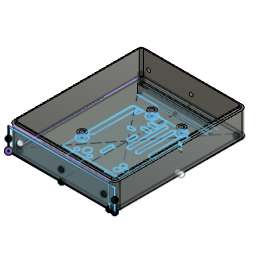
Toolbox-bottom (Autodesk Fusion 360 design; units mm, degrees)
Autodesk Fusion 360 part; units mm, degrees
sketch "Sketch1" plane through (0, 0, 0) normal (0, 1, 0) x (1, 0, 0)
  line L0 (5, 0) -> (95, 0)
  line L1 (100, 5) -> (100, 120)
  line L2 (95, 125) -> (5, 125)
  line L3 (0, 120) -> (0, 5)
  arc A0 (5, 125) -> (0, 120) centre (5, 120) ccw
  arc A1 (100, 120) -> (95, 125) centre (95, 120) ccw
  arc A2 (95, 0) -> (100, 5) centre (95, 5) ccw
  arc A3 (0, 5) -> (5, 0) centre (5, 5) ccw
  line L4 (5, 3) -> (95, 3)
  arc A4 (95, 3) -> (97, 5) centre (95, 5) ccw
  line L5 (97, 5) -> (97, 120)
  arc A5 (97, 120) -> (95, 122) centre (95, 120) ccw
  line L6 (95, 122) -> (5, 122)
  arc A6 (5, 122) -> (3, 120) centre (5, 120) ccw
  line L7 (3, 120) -> (3, 5)
  arc A7 (3, 5) -> (5, 3) centre (5, 5) ccw
  point P0 (100, 0)
  point P1 (0, 125)
  dimension "d1" = 100
  dimension "d2" = 125
  dimension "d5" = -3
  dimension "d9" = 5
  dimension "d10" = 5
  dimension "d11" = 5
  dimension "d12" = 5
  constraint horizontal L0
  constraint vertical L1
  constraint horizontal L2
  constraint vertical L3
  constraint coincident P1 L3
  constraint coincident P1 L2
  constraint tangent L3 A0
  constraint tangent L2 A0
  constraint tangent L2 A1
  constraint tangent L1 A1
  constraint coincident P0 L0
  constraint coincident P0 L1
  constraint tangent L0 A2
  constraint tangent L1 A2
  constraint coincident origin L3
  constraint coincident origin L0
  constraint tangent L3 A3
  constraint tangent L0 A3
  measures "d1" distance of origin P0
  measures "d2" distance of origin P1
  measures "d9" radius of A0
  measures "d10" radius of A1
  measures "d11" radius of A2
  measures "d12" radius of A3
extrude "Extrude1" add sketch "Sketch1" along normal blind 25 contours L0 L1 L2 L3 A0 A1 A2 A3 | L4 A4 L5 A5 L6 A6 L7 A7
extrude "Extrude2" cut sketch "Sketch1" along normal up to surface (23 mm away) from surface at 2 contours L4 A4 L5 A5 L6 A6 L7 A7
ref_plane "WorkPlane1" through (50, 12.5, -62.5) normal (0, 0, 1) x (1, 0, 0)
sketch "Sketch2" plane through (50, 10, -62.5) normal (0, 0, 1) x (1, 0, 0)
ref_plane "WorkPlane2" through (50, 13.5, -64) normal (0, 0, -1) x (-1, 0, 0)
ref_plane "WorkPlane3" through (50, 12.5, -62.5) normal (0, 0, 1) x (1, 0, 0)
sketch "Sketch4" plane through (50, 10, -62.5) normal (0, 0, 1) x (1, 0, 0)
  line L0 (50, 10) -> (50, 8)
  line L1 (50, 8) -> (48, 8)
  line L2 (48, 8) -> (48, 10)
  line L3 (48, 10) -> (50, 10)
  line L4 (50, -10) -> (47, -10)
  line L5 (50, 15) -> (48, 15)
  line L6 (48, 15) -> (48, 13)
  line L7 (48, 13) -> (50, 13)
  line L8 (50, 13) -> (50, 15)
  dimension "d29" = 2
  dimension "d53" = 2
  dimension "d54" = 2
  dimension "d55" = 2
  constraint perpendicular L0 L1
  constraint perpendicular L1 L2
  constraint perpendicular L0 L3
  constraint horizontal L4
  constraint horizontal L5
  constraint vertical L6
  constraint horizontal L7
  constraint vertical L8
  measures "d29" distance of L0 L2
  measures "d53" distance of L1 L3
  measures "d54" distance of L5.start L5.end
  measures "d55" distance of L5.start L7.end
sweep "Sweep1" cut profiles "Sketch4" along 8 edges at (1.4645, 25, -123.5355) (0, 25, -62.5) (1.4645, 25, -1.4645) (50, 25, 0) (98.5355, 25, -1.4645) (100, 25, -62.5) (98.5355, 25, -123.5355) (50, 25, -125) section 1 contours L5 L6 L7 L8
sketch "Sketch5" plane through (0, 0, 0) normal (0, 0, 1) x (1, 0, 0)
  line L0 (5, 23) -> (5, 0)
  line L1 (5, 0) -> (95, 0)
  line L2 (95, 0) -> (95, 23)
  line L3 (0, 0) -> (100, 0)
  line L4 (100, 0) -> (100, 20)
  line L5 (100, 20) -> (0, 20)
  line L6 (0, 20) -> (0, 0)
  circle A0 centre (11, 12) radius 1.75
  line L7 (95, 20) -> (95, 0)
  line L8 (95, 23) -> (5, 23)
  dimension "d19" = 3.5
  constraint horizontal L3
  constraint vertical L4
  constraint horizontal L5
  constraint vertical L6
  constraint coincident L3.start L6.end
  constraint coincident L5 L7.start
  constraint coincident L1.end L2.start
  measures "d19" diameter of A0
sketch "Sketch6" plane through (0, 0, 0) normal (0, 0, 1) x (1, 0, 0)
  line L0 (0, 0) -> (100, 0)
  line L1 (100, 0) -> (100, 20)
  line L2 (100, 20) -> (0, 20)
  line L3 (0, 20) -> (0, 0)
  line L4 (0, 0) -> (100, 0)
  line L5 (0, 0) -> (100, 0)
  line L6 (100, 0) -> (100, 20)
  line L7 (100, 20) -> (0, 20)
  line L8 (0, 20) -> (0, 0)
  circle A0 centre (50, 10) radius 1.75
  circle A1 centre (10, 10) radius 1.75
  circle A2 centre (90, 10) radius 1.75
  point P0 (0, 10)
  point P1 (100, 10)
  point P2 (50, 0)
  dimension "d20" = 20
  dimension "d21" = 100
  dimension "d22" = 3.5
  dimension "d23" = 3.5
  dimension "d24" = 3.5
  dimension "d25" = 10
  dimension "d26" = 10
  constraint horizontal L0
  constraint vertical L1
  constraint horizontal L2
  constraint vertical L3
  constraint coincident L0.start L3.end
  constraint horizontal L5
  constraint vertical L6
  constraint horizontal L7
  constraint vertical L8
  constraint midpoint L3 P0
  constraint midpoint L1 P1
  constraint midpoint L4 P2
  constraint vertical P2 A0.centre
  constraint horizontal P0 A0.centre
  constraint horizontal P0 A1.centre
  constraint horizontal P1 A2.centre
  measures "d20" distance of L1.end L0.end
  measures "d21" distance of L1.end L2.end
  measures "d22" diameter of A0
  measures "d23" diameter of A1
  measures "d24" diameter of A2
  measures "d25" distance of L3 A1.centre
  measures "d26" distance of L1 A2.centre
extrude "Extrude3" cut sketch "Sketch6" against normal up to surface (125 mm away) contours A0 | A1 | A2
sketch "nookduino_holes_thmt_fmsu" plane through (0, 2, 0) normal (0, 1, 0) x (1, 0, 0)
  spline S0 degree 3 poles (36.3365, 93.969) (36.3715, 93.969) (36.3998, 93.9972) (36.3998, 94.0324) (36.3998, 94.0672) (36.3715, 94.0958) (36.3365, 94.0958) knots 0 0 0 0 1 1 1 2 2 2 2
  spline S1 degree 3 poles (23.3685, 92.5565) (23.3437, 92.532) (23.3437, 92.4917) (23.3685, 92.4669) knots 0 0 0 0 1 1 1 1
  spline S2 degree 3 poles (23.3685, 92.4669) (23.3931, 92.4425) (23.4333, 92.4425) (23.4579, 92.4669) knots 1 1 1 1 2 2 2 2
  line L0 (73.3326, 26.3498) -> (73.3326, 28.0274)
  spline S3 degree 3 poles (44.503, 21.7606) (44.5381, 21.7606) (44.5664, 21.789) (44.5664, 21.824) (44.5664, 21.8591) (44.5381, 21.8874) (44.503, 21.8874) knots 0 0 0 0 1 1 1 2 2 2 2
  line L1 (23.4131, 92.5121) -> (24.9336, 94.0324)
  line L2 (38.8704, 96.5663) -> (71.5587, 96.5663)
  spline S4 degree 3 poles (38.617, 39.0459) (40.2416, 39.0459) (41.5581, 37.7292) (41.5581, 36.105) knots 0 0 0 0 1 1 1 1
  line L3 (41.5581, 36.105) -> (41.5581, 35.1974)
  spline S5 degree 3 poles (41.5581, 35.1974) (41.5581, 33.573) (40.2416, 32.2563) (38.617, 32.2563) knots 2 2 2 2 3 3 3 3
  spline S6 degree 3 poles (38.617, 32.2563) (36.9928, 32.2563) (35.6759, 33.573) (35.6759, 35.1974) knots 4 4 4 4 5 5 5 5
  line L4 (35.6759, 35.1974) -> (35.6759, 36.105)
  spline S7 degree 3 poles (35.6759, 36.105) (35.6759, 37.7292) (36.9928, 39.0459) (38.617, 39.0459) knots 6 6 6 6 7 7 7 7
  arc A0 (36.2917, 94.0772) -> (36.2917, 93.9876) centre (36.3364, 94.0324) ccw
  spline S8 degree 3 poles (36.2917, 93.9876) (36.3164, 93.9625) (36.3565, 93.9625) (36.3813, 93.9876) knots 1 1 1 1 2 2 2 2
  spline S9 degree 3 poles (76.5634, 28.149) (76.5634, 28.1141) (76.5916, 28.0856) (76.6264, 28.0856) (76.6616, 28.0856) (76.6898, 28.1141) (76.6898, 28.149) knots 0 0 0 0 1 1 1 2 2 2 2
  spline S10 degree 3 poles (24.9336, 94.0958) (24.8986, 94.0958) (24.8704, 94.0672) (24.8704, 94.0324) (24.8704, 93.9972) (24.8986, 93.969) (24.9336, 93.969) knots 0 0 0 0 1 1 1 2 2 2 2
  line L5 (44.503, 21.824) -> (44.503, 28.0856)
  arc A1 (38.9152, 96.5215) -> (38.9152, 96.611) centre (38.8706, 96.5663) ccw
  spline S11 degree 3 poles (38.9152, 96.611) (38.8906, 96.6358) (38.8504, 96.6358) (38.8258, 96.611) knots 1 1 1 1 2 2 2 2
  spline S12 degree 3 poles (43.0869, 75.547) (43.8496, 75.547) (44.4678, 74.9286) (44.4678, 74.1659) knots 0 0 0 0 1 1 1 1
  spline S13 degree 3 poles (44.4678, 74.1659) (44.4678, 73.4035) (43.8496, 72.7851) (43.0869, 72.7851) knots 2 2 2 2 3 3 3 3
  line L6 (43.0869, 72.7851) -> (40.0261, 72.7851)
  spline S14 degree 3 poles (40.0261, 72.7851) (39.2635, 72.7851) (38.6451, 73.4035) (38.6451, 74.1659) knots 4 4 4 4 5 5 5 5
  spline S15 degree 3 poles (38.6451, 74.1659) (38.6451, 74.9286) (39.2635, 75.547) (40.0261, 75.547) knots 6 6 6 6 7 7 7 7
  line L7 (40.0261, 75.547) -> (43.0869, 75.547)
  line L8 (36.3365, 94.0324) -> (38.8704, 96.5663)
  spline S16 degree 3 poles (76.6898, 94.0324) (76.6898, 94.0672) (76.6616, 94.0958) (76.6264, 94.0958) (76.5916, 94.0958) (76.5634, 94.0672) (76.5634, 94.0324) knots 0 0 0 0 1 1 1 2 2 2 2
  spline S17 degree 3 poles (24.9784, 93.9876) (25.0032, 94.0124) (25.0032, 94.0524) (24.9784, 94.0772) (24.9536, 94.102) (24.9135, 94.102) (24.8888, 94.0772) knots 0 0 0 0 1 1 1 2 2 2 2
  spline S18 degree 3 poles (71.6035, 96.611) (71.579, 96.6358) (71.5387, 96.6358) (71.5139, 96.611) knots 0 0 0 0 1 1 1 1
  spline S19 degree 3 poles (71.5139, 96.611) (71.4895, 96.5862) (71.4895, 96.5463) (71.5139, 96.5215) knots 1 1 1 1 2 2 2 2
  spline S20 degree 3 poles (48.259, 69.3145) (48.259, 70.2171) (48.9907, 70.9489) (49.8933, 70.9489) knots 0 0 0 0 1 1 1 1
  spline S21 degree 3 poles (49.8933, 70.9489) (50.7961, 70.9489) (51.5279, 70.2171) (51.5279, 69.3145) knots 2 2 2 2 3 3 3 3
  line L9 (51.5279, 69.3145) -> (51.5279, 64.2692)
  spline S22 degree 3 poles (51.5279, 64.2692) (51.5279, 63.3665) (50.7961, 62.6348) (49.8933, 62.6348) knots 4 4 4 4 5 5 5 5
  spline S23 degree 3 poles (49.8933, 62.6348) (48.9907, 62.6348) (48.259, 63.3665) (48.259, 64.2692) knots 6 6 6 6 7 7 7 7
  line L10 (48.259, 64.2692) -> (48.259, 69.3145)
  spline S24 degree 3 poles (41.1509, 95.6285) (40.2695, 95.6285) (39.5548, 94.914) (39.5548, 93.1508) (40.2695, 92.4363) (41.1509, 92.4363) (42.0327, 92.4363) (42.7472, 93.1508) (42.7472, 94.914) (42.0327, 95.6285) (41.1509, 95.6285) knots 0 0 0 0 1 1 2 2 2 3 3 4 4 4 4
  line L11 (76.6264, 94.0324) -> (76.6264, 28.149)
  spline S25 degree 3 poles (46.4024, 31.95) (46.4024, 30.9575) (45.5952, 30.1503) (44.6027, 30.1503) (43.6103, 30.1503) (42.803, 30.9575) (42.803, 31.95) (42.803, 32.9424) (43.6103, 33.7497) (44.6027, 33.7497) (45.5952, 33.7497) (46.4024, 32.9424) (46.4024, 31.95) knots 0 0 0 0 1 1 1 2 2 2 3 3 3 4 4 4 4
  spline S26 degree 3 poles (51.0834, 96.5921) (52.5524, 96.5921) (53.7438, 94.9415) (53.7438, 92.9052) knots 0 0 0 0 1 1 1 1
  spline S27 degree 3 poles (53.7438, 92.9052) (53.7438, 90.8684) (52.5524, 89.2179) (51.0834, 89.2179) knots 2 2 2 2 3 3 3 3
  line L12 (51.0834, 89.2179) -> (46.5225, 89.2179)
  spline S28 degree 3 poles (46.5225, 89.2179) (45.053, 89.2179) (43.8618, 90.8684) (43.8618, 92.9052) knots 4 4 4 4 5 5 5 5
  spline S29 degree 3 poles (43.8618, 92.9052) (43.8618, 94.9415) (45.053, 96.5921) (46.5225, 96.5921) knots 6 6 6 6 7 7 7 7
  line L13 (46.5225, 96.5921) -> (51.0834, 96.5921)
  line L14 (71.5587, 96.5663) -> (74.0926, 94.0324)
  line L15 (64.3622, 28.2122) -> (64.3622, 26.3498)
  spline S30 degree 3 poles (23.3499, 28.149) (23.3499, 28.1141) (23.3781, 28.0856) (23.4131, 28.0856) (23.4483, 28.0856) (23.4767, 28.1141) (23.4767, 28.149) knots 0 0 0 0 1 1 1 2 2 2 2
  spline S31 degree 3 poles (64.3305, 26.3498) (64.3305, 26.3323) (64.3447, 26.3183) (64.3622, 26.3183) (64.3798, 26.3183) (64.3936, 26.3323) (64.3936, 26.3498) knots 0 0 0 0 1 1 1 2 2 2 2
  spline S32 degree 3 poles (70.6898, 39.8052) (70.6898, 38.5098) (69.636, 37.456) (68.3406, 37.456) (67.0449, 37.456) (65.9911, 38.5098) (65.9911, 39.8052) (65.9911, 41.1007) (67.0449, 42.1546) (68.3406, 42.1546) (69.636, 42.1546) (70.6898, 41.1007) (70.6898, 39.8052) knots 0 0 0 0 1 1 1 2 2 2 3 3 3 4 4 4 4
  spline S33 degree 3 poles (29.9381, 92.7215) (29.9381, 93.4574) (30.5565, 94.0544) (31.3193, 94.0544) knots 0 0 0 0 1 1 1 1
  spline S34 degree 3 poles (31.3193, 94.0544) (32.0818, 94.0544) (32.7002, 93.4574) (32.7002, 92.7215) knots 2 2 2 2 3 3 3 3
  line L16 (32.7002, 92.7215) -> (32.7002, 89.7687)
  spline S35 degree 3 poles (32.7002, 89.7687) (32.7002, 89.0329) (32.0818, 88.4358) (31.3193, 88.4358) knots 4 4 4 4 5 5 5 5
  spline S36 degree 3 poles (31.3193, 88.4358) (30.5565, 88.4358) (29.9381, 89.0329) (29.9381, 89.7687) knots 6 6 6 6 7 7 7 7
  line L17 (29.9381, 89.7687) -> (29.9381, 92.7215)
  spline S37 degree 3 poles (34.4311, 31.95) (34.4311, 30.9575) (33.6237, 30.1503) (32.6313, 30.1503) (31.6388, 30.1503) (30.8316, 30.9575) (30.8316, 31.95) (30.8316, 32.9424) (31.6388, 33.7497) (32.6313, 33.7497) (33.6237, 33.7497) (34.4311, 32.9424) (34.4311, 31.95) knots 0 0 0 0 1 1 1 2 2 2 3 3 3 4 4 4 4
  spline S38 degree 3 poles (71.5587, 96.5032) (71.5935, 96.5032) (71.6221, 96.5311) (71.6221, 96.5663) (71.6221, 96.6011) (71.5935, 96.6296) (71.5587, 96.6296) knots 0 0 0 0 1 1 1 2 2 2 2
  spline S39 degree 3 poles (75.6821, 36.8152) (75.6821, 35.5196) (74.6283, 34.4656) (73.3326, 34.4656) (72.0369, 34.4656) (70.9834, 35.5196) (70.9834, 36.8152) (70.9834, 38.1105) (72.0369, 39.1646) (73.3326, 39.1646) (74.6283, 39.1646) (75.6821, 38.1105) (75.6821, 36.8152) knots 0 0 0 0 1 1 1 2 2 2 3 3 3 4 4 4 4
  spline S40 degree 3 poles (74.0926, 93.5018) (75.4506, 93.5018) (76.5506, 92.4008) (76.5506, 91.0434) knots 0 0 0 0 1 1 1 1
  line L18 (76.5506, 91.0434) -> (76.5506, 61.5458)
  spline S41 degree 3 poles (76.5506, 61.5458) (76.5506, 60.1877) (75.4506, 59.0874) (74.0926, 59.0874) knots 2 2 2 2 3 3 3 3
  spline S42 degree 3 poles (74.0926, 59.0874) (72.7352, 59.0874) (71.6345, 60.1877) (71.6345, 61.5458) knots 4 4 4 4 5 5 5 5
  line L19 (71.6345, 61.5458) -> (71.6345, 91.0434)
  spline S43 degree 3 poles (71.6345, 91.0434) (71.6345, 92.4008) (72.7352, 93.5018) (74.0926, 93.5018) knots 6 6 6 6 7 7 7 7
  spline S44 degree 3 poles (44.4398, 21.824) (44.4398, 21.789) (44.468, 21.7606) (44.503, 21.7606) (44.5381, 21.7606) (44.5664, 21.789) (44.5664, 21.824) knots 0 0 0 0 1 1 1 2 2 2 2
  spline S45 degree 3 poles (73.3326, 26.3181) (73.3501, 26.3181) (73.3643, 26.3323) (73.3643, 26.3498) (73.3643, 26.3672) (73.3501, 26.3815) (73.3326, 26.3815) knots 0 0 0 0 1 1 1 2 2 2 2
  spline S46 degree 3 poles (64.0835, 92.3853) (65.0533, 92.3853) (65.8395, 91.6587) (65.8395, 90.763) knots 0 0 0 0 1 1 1 1
  line L20 (65.8395, 90.763) -> (65.8395, 58.0249)
  spline S47 degree 3 poles (65.8395, 58.0249) (65.8395, 57.1292) (65.0533, 56.4026) (64.0835, 56.4026) knots 2 2 2 2 3 3 3 3
  spline S48 degree 3 poles (64.0835, 56.4026) (63.1141, 56.4026) (62.3279, 57.1292) (62.3279, 58.0249) knots 4 4 4 4 5 5 5 5
  line L21 (62.3279, 58.0249) -> (62.3279, 90.763)
  spline S49 degree 3 poles (62.3279, 90.763) (62.3279, 91.6587) (63.1141, 92.3853) (64.0835, 92.3853) knots 6 6 6 6 7 7 7 7
  spline S50 degree 3 poles (73.3009, 26.3498) (73.3009, 26.3323) (73.315, 26.3181) (73.3326, 26.3181) (73.3501, 26.3181) (73.3643, 26.3323) (73.3643, 26.3498) knots 0 0 0 0 1 1 1 2 2 2 2
  spline S51 degree 3 poles (74.0481, 93.9876) (74.0726, 93.9625) (74.1129, 93.9625) (74.1374, 93.9876) knots 0 0 0 0 1 1 1 1
  arc A2 (74.1374, 93.9876) -> (74.1374, 94.0772) centre (74.0927, 94.0324) ccw
  spline S52 degree 3 poles (23.4767, 92.5121) (23.4767, 92.5469) (23.4483, 92.5755) (23.4131, 92.5755) (23.3781, 92.5755) (23.3499, 92.5469) (23.3499, 92.5121) knots 0 0 0 0 1 1 1 2 2 2 2
  line L22 (23.4131, 28.149) -> (23.4131, 92.5121)
  spline S53 degree 3 poles (71.3234, 94.0324) (71.3234, 92.7649) (70.2923, 91.7338) (69.0248, 91.7338) (67.7574, 91.7338) (66.7263, 92.7649) (66.7263, 94.0324) (66.7263, 95.2998) (67.7574, 96.331) (69.0248, 96.331) (70.2923, 96.331) (71.3234, 95.2998) (71.3234, 94.0324) knots 0 0 0 0 1 1 1 2 2 2 3 3 3 4 4 4 4
  line L23 (24.9336, 94.0324) -> (36.3365, 94.0324)
  spline S54 degree 3 poles (32.6677, 21.824) (32.6677, 21.789) (32.6961, 21.7606) (32.7311, 21.7606) (32.766, 21.7606) (32.7943, 21.789) (32.7943, 21.824) knots 0 0 0 0 1 1 1 2 2 2 2
  spline S55 degree 3 poles (43.4495, 94.0324) (43.4495, 92.7649) (42.4185, 91.7338) (41.1509, 91.7338) (39.8834, 91.7338) (38.8525, 92.7649) (38.8525, 94.0324) (38.8525, 95.2998) (39.8834, 96.331) (41.1509, 96.331) (42.4185, 96.331) (43.4495, 95.2998) (43.4495, 94.0324) knots 0 0 0 0 1 1 1 2 2 2 3 3 3 4 4 4 4
  spline S56 degree 3 poles (46.8522, 51.7626) (47.7093, 51.7626) (48.4037, 51.0682) (48.4037, 50.2114) knots 0 0 0 0 1 1 1 1
  line L24 (48.4037, 50.2114) -> (48.4037, 42.0691)
  spline S57 degree 3 poles (48.4037, 42.0691) (48.4037, 41.2125) (47.7093, 40.5178) (46.8522, 40.5178) knots 2 2 2 2 3 3 3 3
  spline S58 degree 3 poles (46.8522, 40.5178) (45.9956, 40.5178) (45.3012, 41.2125) (45.3012, 42.0691) knots 4 4 4 4 5 5 5 5
  line L25 (45.3012, 42.0691) -> (45.3012, 50.2114)
  spline S59 degree 3 poles (45.3012, 50.2114) (45.3012, 51.0682) (45.9956, 51.7626) (46.8522, 51.7626) knots 6 6 6 6 7 7 7 7
  spline S60 degree 3 poles (25.9472, 44.949) (25.0656, 44.949) (24.3509, 44.2344) (24.3509, 43.3529) (24.3509, 42.4713) (25.0656, 41.7566) (26.8288, 41.7566) (27.5433, 42.4713) (27.5433, 43.3529) (27.5433, 44.2344) (26.8288, 44.949) (25.9472, 44.949) knots 0 0 0 0 1 1 1 2 2 3 3 3 4 4 4 4
  spline S61 degree 3 poles (23.4131, 28.2122) (23.3781, 28.2122) (23.3499, 28.184) (23.3499, 28.149) (23.3499, 28.1141) (23.3781, 28.0856) (23.4131, 28.0856) knots 0 0 0 0 1 1 1 2 2 2 2
  line L26 (64.3622, 26.3498) -> (73.3326, 26.3498)
  spline S62 degree 3 poles (52.0998, 88.091) (53.0024, 88.091) (53.7341, 87.3589) (53.7341, 86.4566) knots 0 0 0 0 1 1 1 1
  spline S63 degree 3 poles (53.7341, 86.4566) (53.7341, 85.554) (53.0024, 84.8219) (52.0998, 84.8219) knots 2 2 2 2 3 3 3 3
  line L27 (52.0998, 84.8219) -> (47.0546, 84.8219)
  spline S64 degree 3 poles (47.0546, 84.8219) (46.152, 84.8219) (45.4202, 85.554) (45.4202, 86.4566) knots 4 4 4 4 5 5 5 5
  spline S65 degree 3 poles (45.4202, 86.4566) (45.4202, 87.3589) (46.152, 88.091) (47.0546, 88.091) knots 6 6 6 6 7 7 7 7
  line L28 (47.0546, 88.091) -> (52.0998, 88.091)
  spline S66 degree 3 poles (28.2457, 43.3529) (28.2457, 42.0853) (27.2146, 41.0544) (25.9472, 41.0544) (24.6797, 41.0544) (23.6486, 42.0853) (23.6486, 43.3529) (23.6486, 44.6204) (24.6797, 45.6513) (25.9472, 45.6513) (27.2146, 45.6513) (28.2457, 44.6204) (28.2457, 43.3529) knots 0 0 0 0 1 1 1 2 2 2 3 3 3 4 4 4 4
  spline S67 degree 3 poles (38.8704, 96.6296) (38.8354, 96.6296) (38.8072, 96.6011) (38.8072, 96.5663) (38.8072, 96.5311) (38.8354, 96.5032) (38.8704, 96.5032) knots 0 0 0 0 1 1 1 2 2 2 2
  spline S68 degree 3 poles (76.6264, 28.0856) (76.6616, 28.0856) (76.6898, 28.1141) (76.6898, 28.149) (76.6898, 28.184) (76.6616, 28.2122) (76.6264, 28.2122) knots 0 0 0 0 1 1 1 2 2 2 2
  spline S69 degree 3 poles (52.0998, 81.6039) (53.0024, 81.6039) (53.7341, 80.8721) (53.7341, 79.9695) knots 0 0 0 0 1 1 1 1
  spline S70 degree 3 poles (53.7341, 79.9695) (53.7341, 79.0669) (53.0024, 78.3351) (52.0998, 78.3351) knots 2 2 2 2 3 3 3 3
  line L29 (52.0998, 78.3351) -> (47.0546, 78.3351)
  spline S71 degree 3 poles (47.0546, 78.3351) (46.152, 78.3351) (45.4202, 79.0669) (45.4202, 79.9695) knots 4 4 4 4 5 5 5 5
  spline S72 degree 3 poles (45.4202, 79.9695) (45.4202, 80.8721) (46.152, 81.6039) (47.0546, 81.6039) knots 6 6 6 6 7 7 7 7
  line L30 (47.0546, 81.6039) -> (52.0998, 81.6039)
  line L31 (76.6264, 28.149) -> (23.4131, 28.149)
  spline S73 degree 3 poles (69.0248, 95.6285) (68.1432, 95.6285) (67.4287, 94.914) (67.4287, 93.1508) (68.1432, 92.4363) (69.9064, 92.4363) (70.6209, 93.1508) (70.6209, 94.914) (69.9064, 95.6285) (69.0248, 95.6285) knots 0 0 0 0 1 1 2 2 3 3 4 4 4 4
  spline S74 degree 3 poles (70.6898, 33.8252) (70.6898, 32.5296) (69.636, 31.4756) (68.3406, 31.4756) (67.0449, 31.4756) (65.9911, 32.5296) (65.9911, 33.8252) (65.9911, 35.1205) (67.0449, 36.1746) (68.3406, 36.1746) (69.636, 36.1746) (70.6898, 35.1205) (70.6898, 33.8252) knots 0 0 0 0 1 1 1 2 2 2 3 3 3 4 4 4 4
  spline S75 degree 3 poles (25.9473, 93.681) (27.305, 93.681) (28.4054, 92.5806) (28.4054, 91.2229) knots 0 0 0 0 1 1 1 1
  line L32 (28.4054, 91.2229) -> (28.4054, 52.2435)
  spline S76 degree 3 poles (28.4054, 52.2435) (28.4054, 50.886) (27.305, 49.7854) (25.9473, 49.7854) knots 2 2 2 2 3 3 3 3
  spline S77 degree 3 poles (25.9473, 49.7854) (24.5896, 49.7854) (23.4892, 50.886) (23.4892, 52.2435) knots 4 4 4 4 5 5 5 5
  line L33 (23.4892, 52.2435) -> (23.4892, 91.2229)
  spline S78 degree 3 poles (23.4892, 91.2229) (23.4892, 92.5806) (24.5896, 93.681) (25.9473, 93.681) knots 6 6 6 6 7 7 7 7
  spline S79 degree 3 poles (32.7311, 21.8874) (32.6961, 21.8874) (32.6677, 21.8591) (32.6677, 21.824) (32.6677, 21.789) (32.6961, 21.7606) (32.7311, 21.7606) knots 0 0 0 0 1 1 1 2 2 2 2
  spline S80 degree 3 poles (56.4816, 92.695) (57.4514, 92.695) (58.2372, 92.0105) (58.2372, 91.1664) knots 0 0 0 0 1 1 1 1
  line L34 (58.2372, 91.1664) -> (58.2372, 57.6215)
  spline S81 degree 3 poles (58.2372, 57.6215) (58.2372, 56.7771) (57.4514, 56.0926) (56.4816, 56.0926) knots 2 2 2 2 3 3 3 3
  spline S82 degree 3 poles (56.4816, 56.0926) (55.5118, 56.0926) (54.7256, 56.7771) (54.7256, 57.6215) knots 4 4 4 4 5 5 5 5
  line L35 (54.7256, 57.6215) -> (54.7256, 91.1664)
  spline S83 degree 3 poles (54.7256, 91.1664) (54.7256, 92.0105) (55.5118, 92.695) (56.4816, 92.695) knots 6 6 6 6 7 7 7 7
  spline S84 degree 3 poles (74.0926, 94.0958) (74.0578, 94.0958) (74.0295, 94.0672) (74.0295, 94.0324) (74.0295, 93.9972) (74.0578, 93.969) (74.0926, 93.969) knots 0 0 0 0 1 1 1 2 2 2 2
  line L36 (74.0926, 94.0324) -> (76.6264, 94.0324)
  spline S85 degree 3 poles (64.3622, 26.3815) (64.3447, 26.3815) (64.3305, 26.3672) (64.3305, 26.3498) (64.3305, 26.3323) (64.3447, 26.3181) (64.3622, 26.3181) knots 0 0 0 0 1 1 1 2 2 2 2
  line L37 (32.7311, 21.824) -> (44.503, 21.824)
  spline S86 degree 3 poles (76.6264, 93.969) (76.6616, 93.969) (76.6898, 93.9972) (76.6898, 94.0324) (76.6898, 94.0672) (76.6616, 94.0958) (76.6264, 94.0958) knots 0 0 0 0 1 1 1 2 2 2 2
  line L38 (32.7311, 28.149) -> (32.7311, 21.824)
  spline S87 degree 3 poles (25.9472, 46.949) (24.6384, 46.949) (23.4669, 46.235) (22.8425, 45.1684) (22.5307, 44.6357) (22.3509, 44.0067) (22.3509, 43.3529) (22.3509, 42.0445) (23.0646, 40.8732) (24.1308, 40.2488) (24.6637, 39.9366) (25.2931, 39.7566) (25.9472, 39.7566) (27.2544, 39.7566) (28.4249, 40.4693) (29.0496, 41.5339) (29.3628, 42.0675) (29.5433, 42.6978) (29.5433, 43.3529) (29.5433, 44.6619) (28.8289, 45.8337) (27.7618, 46.4579) (27.2293, 46.7695) (26.6005, 46.949) (25.9472, 46.949) knots 0 0 0 0 0.666882 0.666882 0.666882 1 1 1 1.666704 1.666704 1.666704 2 2 2 2.666128 2.666128 2.666128 3 3 3 3.66706 3.66706 3.66706 4 4 4 4
  spline S88 degree 3 poles (41.1509, 97.6285) (39.8419, 97.6285) (38.6702, 96.9141) (38.0459, 95.8471) (37.7343, 95.3145) (37.5548, 94.6858) (37.5548, 94.0324) (37.5548, 92.7248) (38.2678, 91.5541) (39.3328, 90.9294) (39.8661, 90.6166) (40.4961, 90.4363) (41.1509, 90.4363) (42.4587, 90.4363) (43.6299, 91.1494) (44.2545, 92.215) (44.567, 92.7482) (44.7472, 93.3779) (44.7472, 94.0324) (44.7472, 95.3398) (44.0343, 96.5107) (42.9691, 97.1354) (42.4357, 97.4482) (41.8057, 97.6285) (41.1509, 97.6285) knots 0 0 0 0 0.66706 0.66706 0.66706 1 1 1 1.666306 1.666306 1.666306 2 2 2 2.666482 2.666482 2.666482 3 3 3 3.666305 3.666305 3.666305 4 4 4 4
  spline S89 degree 3 poles (69.0248, 97.6285) (67.717, 97.6285) (66.5459, 96.9153) (65.9214, 95.8497) (65.6088, 95.3165) (65.4287, 94.6868) (65.4287, 94.0324) (65.4287, 92.7246) (66.1419, 91.5535) (67.2075, 90.9289) (67.7407, 90.6164) (68.3704, 90.4363) (69.0248, 90.4363) (70.3326, 90.4363) (71.5037, 91.1495) (72.1283, 92.215) (72.4408, 92.7483) (72.6209, 93.3779) (72.6209, 94.0324) (72.6209, 95.3402) (71.9077, 96.5113) (70.8422, 97.1358) (70.309, 97.4484) (69.6793, 97.6285) (69.0248, 97.6285) knots 0 0 0 0 0.666483 0.666483 0.666483 1 1 1 1.666483 1.666483 1.666483 2 2 2 2.666483 2.666483 2.666483 3 3 3 3.666483 3.666483 3.666483 4 4 4 4
  spline S90 degree 3 poles (25.9472, 47.949) (24.5153, 47.949) (23.1988, 47.2738) (22.3591, 46.2254) (21.731, 45.4413) (21.3509, 44.424) (21.3509, 43.3529) (21.3509, 41.9211) (22.0261, 40.6046) (23.0745, 39.7649) (23.8587, 39.1367) (24.876, 38.7566) (25.9472, 38.7566) (27.3781, 38.7566) (28.694, 39.4312) (29.5336, 40.4784) (30.1627, 41.263) (30.5433, 42.2811) (30.5433, 43.3529) (30.5433, 44.7855) (29.8673, 46.1027) (28.8179, 46.9424) (28.034, 47.5696) (27.0174, 47.949) (25.9472, 47.949) knots 0 0 0 0 0.572087 0.572087 0.572087 1 1 1 1.572058 1.572058 1.572058 2 2 2 2.571697 2.571697 2.571697 3 3 3 3.572422 3.572422 3.572422 4 4 4 4
  spline S91 degree 3 poles (41.1509, 98.6285) (39.7183, 98.6285) (38.4012, 97.9525) (37.5615, 96.9031) (36.9342, 96.1192) (36.5548, 95.1026) (36.5548, 94.0324) (36.5548, 92.6014) (37.2293, 91.2855) (38.2766, 90.4458) (39.0611, 89.8169) (40.079, 89.4363) (41.1509, 89.4363) (42.5832, 89.4363) (43.9006, 90.1121) (44.7404, 91.1615) (45.3678, 91.9456) (45.7472, 92.9623) (45.7472, 94.0324) (45.7472, 95.4643) (45.0717, 96.7813) (44.0228, 97.621) (43.2385, 98.2488) (42.2214, 98.6285) (41.1509, 98.6285) knots 0 0 0 0 0.572422 0.572422 0.572422 1 1 1 1.571726 1.571726 1.571726 2 2 2 2.572386 2.572386 2.572386 3 3 3 3.572194 3.572194 3.572194 4 4 4 4
  spline S92 degree 3 poles (69.0248, 98.6285) (67.5928, 98.6285) (66.2758, 97.953) (65.4361, 96.9041) (64.8084, 96.1199) (64.4287, 95.1029) (64.4287, 94.0324) (64.4287, 92.6004) (65.1042, 91.2834) (66.1532, 90.4437) (66.9373, 89.816) (67.9543, 89.4363) (69.0248, 89.4363) (70.4568, 89.4363) (71.7738, 90.1118) (72.6135, 91.1607) (73.2413, 91.9448) (73.6209, 92.9619) (73.6209, 94.0324) (73.6209, 95.4644) (72.9454, 96.7814) (71.8965, 97.6211) (71.1124, 98.2488) (70.0954, 98.6285) (69.0248, 98.6285) knots 0 0 0 0 0.572223 0.572223 0.572223 1 1 1 1.572223 1.572223 1.572223 2 2 2 2.572223 2.572223 2.572223 3 3 3 3.572223 3.572223 3.572223 4 4 4 4
  line L39 (17.7, 114) -> (83.7, 114)
  line L40 (3, 5) -> (3, 120)
  spline S93 degree 3 poles (25.9472, 45.449) (24.7953, 45.449) (23.8509, 44.5046) (23.8509, 43.3529) (23.8509, 42.2011) (24.7953, 41.2566) (25.9472, 41.2566) (27.099, 41.2566) (28.0433, 42.2012) (28.0433, 43.3529) (28.0433, 44.5046) (27.099, 45.449) (25.9472, 45.449) knots 0 0 0 0 1 1 1 2 2 2 3 3 3 4 4 4 4
  spline S94 degree 3 poles (69.0248, 96.1285) (67.8731, 96.1285) (66.9287, 95.1841) (66.9287, 94.0324) (66.9287, 92.8806) (67.8731, 91.9363) (69.0248, 91.9363) (70.1766, 91.9363) (71.1209, 92.8806) (71.1209, 94.0324) (71.1209, 95.1841) (70.1766, 96.1285) (69.0248, 96.1285) knots 0 0 0 0 1 1 1 2 2 2 3 3 3 4 4 4 4
  spline S95 degree 3 poles (41.1509, 96.1285) (39.9992, 96.1285) (39.0548, 95.1842) (39.0548, 94.0324) (39.0548, 92.8806) (39.9992, 91.9363) (41.1509, 91.9363) (42.3028, 91.9363) (43.2472, 92.8806) (43.2472, 94.0324) (43.2472, 95.1841) (42.3028, 96.1285) (41.1509, 96.1285) knots 0 0 0 0 1 1 1 2 2 2 3 3 3 4 4 4 4
  dimension "d32" = 2
  dimension "d33" = 2
  dimension "d34" = 2
  dimension "d35" = 3
  dimension "d36" = 3
  dimension "d37" = 3
  dimension "d38" = 66
  dimension "d39" = 14.7
  dimension "d46" = 0.5
  dimension "d48" = 0.5
  dimension "d49" = 0.5
  constraint horizontal L39
  measures "d38" distance of L39.start L39.end
  measures "d39" distance of L39.start L40
extrude "Extrude4" add sketch "nookduino_holes_thmt_fmsu" along normal blind 5 contours L2 A1 S11 L8 S67 S88 | L2 L8 S28 S29 S88 | L2 A1 S11 L8 S67 | S28 S29 S88 | L2 S18 S19 S89 | L2 L14 S43 S89 | L2 S18 S19 L14 S38 S89 | S43 S89 | L14 S38 S89 | L22 S87 | L22 S87 | S24 | S53 | S55 | S60 | S66 | S73 | S93 | S94 | S95
sketch "Sketch9" plane through (0, 2, 0) normal (0, 1, 0) x (-1, 0, 0)
  arc A0 (-3, -5) -> (-5, -3) centre (-5, -5) ccw
  line L0 (-5, -3) -> (-95, -3)
  arc A1 (-95, -3) -> (-97, -5) centre (-95, -5) ccw
  line L1 (-97, -5) -> (-97, -120)
  arc A2 (-97, -120) -> (-95, -122) centre (-95, -120) ccw
  line L2 (-95, -122) -> (-5, -122)
  arc A3 (-5, -122) -> (-3, -120) centre (-5, -120) ccw
  line L3 (-3, -120) -> (-3, -5)
  line L4 (-3.5858, -121.4142) -> (-96.4142, -3.5858) construction
  line L5 (-3.5858, -3.5858) -> (-96.4142, -121.4142) construction
  line L6 (-50, -122) -> (-50, -3) construction
  line L7 (-82, -108.0854) -> (-18, -108.0854)
  line L8 (-18, -108.0854) -> (-18, -105.8854)
  line L9 (-18, -105.8854) -> (-82, -105.8854)
  line L10 (-82, -105.8854) -> (-82, -108.0854)
  line L11 (-82, -108.0854) -> (-18, -105.8854) construction
  line L12 (-18, -108.0854) -> (-82, -105.8854) construction
  line L13 (-16.8, -104.6854) -> (-83.2, -104.6854)
  line L14 (-83.2, -104.6854) -> (-83.2, -109.2854)
  line L15 (-83.2, -109.2854) -> (-16.8, -109.2854)
  line L16 (-16.8, -109.2854) -> (-16.8, -104.6854)
  spline S0 degree 3 poles (-69.0248, -97.6285) (-69.6793, -97.6285) (-70.309, -97.4484) (-70.8422, -97.1358) (-71.9077, -96.5113) (-72.6209, -95.3402) (-72.6209, -94.0324) (-72.6209, -93.3779) (-72.4408, -92.7483) (-72.1283, -92.215) (-71.5037, -91.1495) (-70.3326, -90.4363) (-69.0248, -90.4363) (-68.3704, -90.4363) (-67.7407, -90.6164) (-67.2075, -90.9289) (-66.1419, -91.5535) (-65.4287, -92.7246) (-65.4287, -94.0324) (-65.4287, -94.6868) (-65.6088, -95.3165) (-65.9214, -95.8497) (-66.5459, -96.9153) (-67.717, -97.6285) (-69.0248, -97.6285) knots -4 -4 -4 -4 -3.666483 -3.666483 -3.666483 -3 -3 -3 -2.666483 -2.666483 -2.666483 -2 -2 -2 -1.666483 -1.666483 -1.666483 -1 -1 -1 -0.666483 -0.666483 -0.666483 0 0 0 0
  spline S1 degree 3 poles (-41.1509, -97.6285) (-41.8057, -97.6285) (-42.4357, -97.4482) (-42.9691, -97.1354) (-44.0343, -96.5107) (-44.7472, -95.3398) (-44.7472, -94.0324) (-44.7472, -93.3779) (-44.567, -92.7482) (-44.2545, -92.215) (-43.6299, -91.1494) (-42.4587, -90.4363) (-41.1509, -90.4363) (-40.4961, -90.4363) (-39.8661, -90.6166) (-39.3328, -90.9294) (-38.2678, -91.5541) (-37.5548, -92.7248) (-37.5548, -94.0324) (-37.5548, -94.6858) (-37.7343, -95.3145) (-38.0459, -95.8471) (-38.6702, -96.9141) (-39.8419, -97.6285) (-41.1509, -97.6285) knots -4 -4 -4 -4 -3.666305 -3.666305 -3.666305 -3 -3 -3 -2.666482 -2.666482 -2.666482 -2 -2 -2 -1.666306 -1.666306 -1.666306 -1 -1 -1 -0.66706 -0.66706 -0.66706 0 0 0 0
  spline S2 degree 3 poles (-25.9472, -46.949) (-26.6005, -46.949) (-27.2293, -46.7695) (-27.7618, -46.4579) (-28.8289, -45.8337) (-29.5433, -44.6619) (-29.5433, -43.3529) (-29.5433, -42.6978) (-29.3628, -42.0675) (-29.0496, -41.5339) (-28.4249, -40.4693) (-27.2544, -39.7566) (-25.9472, -39.7566) (-25.2931, -39.7566) (-24.6637, -39.9366) (-24.1308, -40.2488) (-23.0646, -40.8732) (-22.3509, -42.0445) (-22.3509, -43.3529) (-22.3509, -44.0067) (-22.5307, -44.6357) (-22.8425, -45.1684) (-23.4669, -46.235) (-24.6384, -46.949) (-25.9472, -46.949) knots -4 -4 -4 -4 -3.66706 -3.66706 -3.66706 -3 -3 -3 -2.666128 -2.666128 -2.666128 -2 -2 -2 -1.666704 -1.666704 -1.666704 -1 -1 -1 -0.666882 -0.666882 -0.666882 0 0 0 0
  point P0 (-50, -106.9854)
  dimension "d40" = 64
  dimension "d41" = 2.2
  dimension "d42" = 1.2
  constraint midpoint A3 L4.start
  constraint midpoint A1 L4.end
  constraint midpoint A0 L5.start
  constraint midpoint A2 L5.end
  constraint midpoint L2 L6.start
  constraint midpoint L0 L6.end
  constraint horizontal L7
  constraint perpendicular L7 L8
  constraint parallel L7 L9
  constraint parallel L8 L10
  constraint coincident L11 P0
  constraint coincident L12 P0
  constraint coincident L6 P0
  measures "d40" distance of L8.end L9.end
  measures "d41" distance of L7.end L8.end
extrude "Extrude5" add sketch "Sketch9" along normal blind 9 contours L13 L14 L15 L16
fillet "Fillet1" radius 4 2 edges at (18, 2, -106.9854) (82, 2, -106.9854)
extrude "Extrude6" cut sketch "nookduino_holes_thmt_fmsu" against normal blind 3.3 from surface at 5 contours S24 | S60 | S73 | S93 | S94 | S95
equation "d26 = d25"
